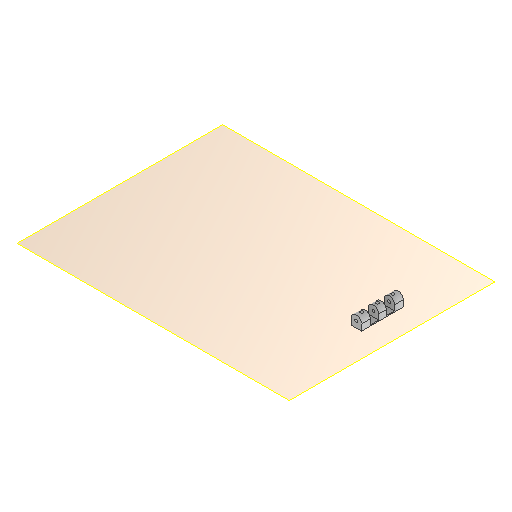
# Autodesk Inventor part: 60_Planktoscope_Illuminationsource
Saved by Autodesk Inventor 2024.1 (Build 281209000, 209)
## iProperties
Created: 2024-07-24
Part Number: 60_Planktoscope_Illuminationsource
Material: Generisch
Document SubType Name: Modeling
Designer: diederichbenedict
Density: 1 g/cm^3
Appearance: Vorgabe
Vendor: openUC2
Mass: 2.23618 g
Surface Area: 21.4305 cm^2
Volume: 2.23618 cm^3
Author: diederichbenedict
Autodesk Inventor part; units mm, degrees
ref_plane "YZ Plane" through (0, 0, 0) normal (1, 0, 0) x (0, 1, 0)
ref_plane "XZ Plane" through (0, 0, 0) normal (0, 1, 0) x (-1, 0, 0)
ref_plane "XY Plane" through (0, 0, 0) normal (0, 0, 1) x (1, 0, 0)
ref_plane "Arbeitsebene1" through (0, 0, 0) normal (0, 0, 1) x (1, 0, 0)
sketch "Skizze1" plane through (0, 0, 0) normal (0, 0, 1) x (1, 0, 0)
  line L0 (-118.5, -74.5) -> (-118.5, 74.5) projected
  arc A0 (-118.5, -74.5) -> (-103.5, -89.5) centre (-103.5, -74.5) ccw projected
  line L1 (56.1, -89.5) -> (-103.5, -89.5) projected
  line L2 (56.1, -83) -> (56.1, -89.5) projected
  arc A1 (71.1, -68) -> (56.1, -83) centre (71.1, -83) ccw projected
  line L3 (80.5, -68) -> (71.1, -68) projected
  arc A2 (95.5, -83) -> (80.5, -68) centre (80.5, -83) ccw projected
  line L4 (95.5, -89.5) -> (95.5, -83) projected
  line L5 (103.5, -89.5) -> (95.5, -89.5) projected
  arc A3 (103.5, -89.5) -> (118.5, -74.5) centre (103.5, -74.5) ccw projected
  line L6 (118.5, 74.5) -> (118.5, -74.5) projected
  arc A4 (118.5, 74.5) -> (103.5, 89.5) centre (103.5, 74.5) ccw projected
  line L7 (-103.5, 89.5) -> (103.5, 89.5) projected
  arc A5 (-103.5, 89.5) -> (-118.5, 74.5) centre (-103.5, 74.5) ccw projected
  circle A6 centre (-58.5, 18.7) radius 1.4 projected
  circle A7 centre (-58.5, 36.552) radius 1.4 projected
  circle A8 centre (57.5, 20.252) radius 1.4 projected
  circle A9 centre (57.5, 35) radius 1.4 projected
  circle A10 centre (-58.5, 8.7) radius 1.4 projected
  circle A11 centre (-58.5, -9.152) radius 1.4 projected
  circle A12 centre (57.5, 7.148) radius 1.4 projected
  circle A13 centre (57.5, -7.6) radius 1.4 projected
  circle A14 centre (103.5, 74.5) radius 1.4 projected
  circle A15 centre (103.5, -74.5) radius 1.4 projected
  circle A16 centre (-103.5, -74.5) radius 1.4 projected
  circle A17 centre (-103.5, 74.5) radius 1.4 projected
  line L8 (20.9567, 0.5738) -> (-20.9567, 0.5738) projected
  line L9 (-20.9567, 0.5738) -> (-20.9567, 30.6837) projected
  line L10 (-20.9567, 30.6837) -> (20.9567, 30.6837) projected
  line L11 (20.9567, 30.6837) -> (20.9567, 0.5738) projected
  circle A18 centre (73.1917, -22.4328) radius 1.4 projected
  circle A19 centre (43.1917, -22.4328) radius 1.4 projected
  circle A20 centre (13.1917, -22.4328) radius 1.4 projected
  circle A21 centre (-16.8083, -22.4328) radius 1.4 projected
  circle A22 centre (-46.8083, -22.4328) radius 1.4 projected
  circle A23 centre (-102.338, -1.3) radius 1.4 projected
  circle A24 centre (-102.338, 13.7) radius 1.4 projected
  circle A25 centre (-102.338, 28.7) radius 1.4 projected
  circle A26 centre (102.338, 28.7) radius 1.4 projected
  circle A27 centre (-73.1917, -22.4328) radius 1.4 projected
  circle A28 centre (-43.1917, -22.4328) radius 1.4 projected
  circle A29 centre (-13.1917, -22.4328) radius 1.4 projected
  circle A30 centre (16.8083, -22.4328) radius 1.4 projected
  circle A31 centre (46.8083, -22.4328) radius 1.4 projected
  circle A32 centre (102.338, -1.3) radius 1.4 projected
  circle A33 centre (102.338, 13.7) radius 1.4 projected
  line L12 (97.338, -6.3) -> (107.338, -6.3)
  line L13 (107.338, -6.3) -> (107.338, 33.7)
  line L14 (107.338, 33.7) -> (97.338, 33.7)
  line L15 (97.338, 33.7) -> (97.338, -6.3)
  line L16 (97.338, -6.3) -> (107.338, 33.7) construction
  line L17 (107.338, -6.3) -> (97.338, 33.7) construction
  line L18 (76.5043, -50) -> (76.5043, 50) projected
  arc A34 (96.5043, 50) -> (76.5043, 50) centre (86.5043, 50) ccw projected
  line L19 (96.5043, 50) -> (96.5043, -50) projected
  arc A35 (76.5043, -50) -> (96.5043, -50) centre (86.5043, -50) ccw projected
  line L20 (-95.8131, -50) -> (-95.8131, 50) projected
  arc A36 (-75.8131, 50) -> (-95.8131, 50) centre (-85.8131, 50) ccw projected
  line L21 (-75.8131, 50) -> (-75.8131, -50) projected
  arc A37 (-95.8131, -50) -> (-75.8131, -50) centre (-85.8131, -50) ccw projected
  circle A38 centre (-108.5, 79.5) radius 1.4 projected
  circle A39 centre (-108.5, -79.5) radius 1.4 projected
  circle A40 centre (108.5, 79.5) radius 1.4 projected
  circle A41 centre (108.5, -79.5) radius 1.4 projected
  point P0 (0, 0)
  dimension "d0" = 10
  dimension "d1" = 40
  constraints: 12 end point, 2 midpoint, 2 parallel, 1 horizontal, 1 perpendicular
  measures "d0" distance of L14.end L13.end
  measures "d1" distance of L13.end L12.end
extrude "Extrusion1" add sketch "Skizze1" along normal blind 50 contours L15 L14 L13 L12
fillet "Rundung1" radius 5 2 edges at (102.338, -6.3, 50) (102.338, 33.7, 50)
sketch "Skizze2" plane through (97.338, 33.7, 0) normal (0, 1, 0) x (1, 0, 0)
  line L0 (10, -45) -> (0, -45) projected
  line L1 (10, 0) -> (10, -45) projected
  line L2 (10, 0) -> (0, 0) projected
  line L3 (0, 0) -> (0, -45) projected
  circle A0 centre (5, -6) radius 5
  line L4 (10, 0) -> (10, -45) projected
  circle A1 centre (5, -6) radius 1.4
  point P0 (-97.338, 0)
  point P1 (0, -6)
  point P2 (10, -6)
  dimension "d5" = 6
  dimension "d8" = 2.8
  constraints: 2 centre point, 1 coincident, 1 tangent
  measures "d5" distance from line of A0.centre L2
  measures "d8" diameter of A1
extrude "Extrusion2" cut sketch "Skizze2" against normal through all contours A0 L3 L2 L1 | A0 keep common part
sketch "Skizze3" plane through (107.338, -6.3, 0) normal (1, 0, 0) x (0, 0, -1)
  line L0 (0, 40) -> (-6, 40) projected
  line L1 (0, 0) -> (-6, 0) projected
  line L2 (-4.6, 33.6) -> (0, 33.6) projected
  line L3 (-4.6, 21.4) -> (0, 21.4) projected
  line L4 (-4.6, 18.6) -> (0, 18.6) projected
  line L5 (-4.6, 6.4) -> (0, 6.4) projected
  line L6 (-4.6, 3.6) -> (0, 3.6) projected
  line L7 (-4.6, 36.4) -> (0, 36.4) projected
  line L8 (-11, 40) -> (-11, 0) projected
  line L9 (-11, 31.6) -> (-1, 31.6)
  line L10 (-1, 31.6) -> (-1, 23.6)
  line L11 (-1, 23.6) -> (-11, 23.6)
  line L12 (-11, 23.6) -> (-11, 31.6)
  line L13 (-11, 16.4) -> (-1, 16.4)
  line L14 (-1, 16.4) -> (-1, 8.4)
  line L15 (-1, 8.4) -> (-11, 8.4)
  line L16 (-11, 8.4) -> (-11, 16.4)
  point P0 (0, 6.3)
  point P1 (-11, 8.4)
  point P2 (-11, 23.6)
  dimension "d9" = 10
  dimension "d10" = 8
  dimension "d11" = 10
  dimension "d12" = 8
  dimension "d13" = 2
  dimension "d14" = 2.2
  constraints: 16 end point, 4 parallel, 2 horizontal, 2 perpendicular, 2 point on line
  measures "d9" distance of L10.end L11.end
  measures "d10" distance of L9.end L10.end
  measures "d11" distance of L14.end L15.end
  measures "d12" distance of L13.end L14.end
  measures "d13" distance between parallel lines of L9 L2
  measures "d14" distance between parallel lines of L13 L4
extrude "Extrusion3" cut sketch "Skizze3" against normal blind 10
